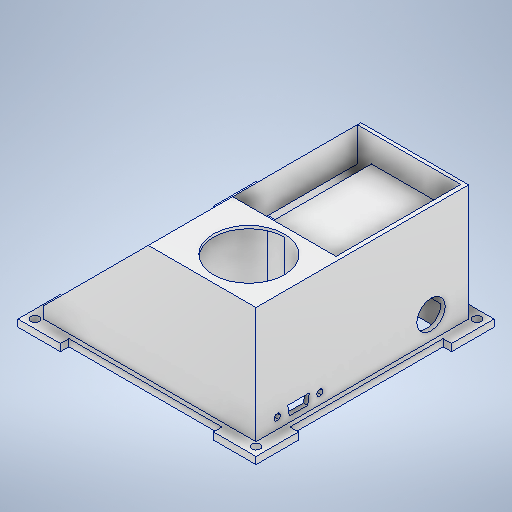
# Autodesk Inventor part: upper half second trial
Saved by Autodesk Inventor 2025 (Build 290162000, 162)
## iProperties
Created: 2024-04-12
Part Number: upper half second trial
Material: Aluminum 6061
Document SubType Name: Modeling
Designer: mahal
Density: 2.7 g/cm^3
Appearance: Aluminum - Flat
Mass: 980.83 g
Surface Area: 1659.79 cm^2
Volume: 363.27 cm^3
Author: mahal
Autodesk Inventor part; units mm, degrees
sketch "Sketch1" plane through (0, 0, 0) normal (0, 1, 0) x (-1, 0, 0)
  line L0 (75, 75) -> (-75, 75)
  line L1 (-75, 75) -> (-75, -75)
  line L2 (-75, -75) -> (75, -75)
  line L3 (75, -75) -> (75, 75)
  line L4 (75, 75) -> (-75, -75) construction
  line L5 (-75, 75) -> (75, -75) construction
  point P0 (0, 0)
  dimension "d0" = 150
  dimension "d1" = 150
  constraints: 12 end point, 2 midpoint, 2 parallel, 1 horizontal, 1 perpendicular
  measures "d0" distance of L2.end L1.end
  measures "d1" distance of L1.end L0.end
extrude "Extrusion1" add sketch "Sketch1" along normal blind 110
ref_plane "Work Plane1" through (0, 0, 0) normal (0, -1, 0) x (1, 0, 0)
sketch "Sketch2" plane through (0, 0, 0) normal (0, -1, 0) x (1, 0, 0)
  line L0 (72, 72) -> (-72, 72)
  line L1 (-72, 72) -> (-72, -72)
  line L2 (-72, -72) -> (72, -72)
  line L3 (72, -72) -> (72, 72)
  line L4 (72, 72) -> (-72, -72) construction
  line L5 (-72, 72) -> (72, -72) construction
  line L6 (72, 72) -> (3, 72)
  line L7 (3, 72) -> (3, 18)
  line L8 (3, 18) -> (72, 18)
  line L9 (72, 18) -> (72, 72)
  line L10 (72, 18) -> (3, 18)
  line L11 (3, 18) -> (3, 14)
  line L12 (3, 14) -> (72, 14)
  line L13 (72, 14) -> (72, 18)
  point P0 (0, 0)
  dimension "d5" = 144
  dimension "d6" = 144
  dimension "d7" = 69
  dimension "d8" = 54
  dimension "d9" = 4
  constraints: 28 end point, 6 parallel, 3 horizontal, 3 perpendicular, 2 midpoint
  measures "d5" distance of L2.end L1.end
  measures "d6" distance of L1.end L0.end
  measures "d7" distance of L8.end L7.end
  measures "d8" distance of L7.end L6.end
  measures "d9" distance of L11.end L10.end
extrude "Extrusion2" cut sketch "Sketch2" against normal blind 5 contours L3 L8 L7 L0
ref_plane "Work Plane2" through (0, 5, 0) normal (0, -1, 0) x (1, 0, 0)
sketch "Sketch4" plane through (0, 5, 0) normal (0, -1, 0) x (1, 0, 0)
  line L0 (72, 18) -> (3, 18)
  line L1 (3, 18) -> (3, 72)
  line L2 (3, 72) -> (72, 72)
  line L3 (72, 72) -> (72, 18)
  line L4 (72, 18) -> (67, 18)
  line L5 (67, 18) -> (67, 25)
  line L6 (67, 25) -> (72, 25)
  line L7 (72, 25) -> (72, 18)
  line L8 (72, 72) -> (67, 72)
  line L9 (67, 72) -> (67, 65)
  line L10 (67, 65) -> (72, 65)
  line L11 (72, 72) -> (72, 65)
  line L12 (67, 18) -> (13, 18)
  line L13 (13, 18) -> (13, 72)
  line L14 (67, 72) -> (13, 72)
  point P0 (0, 0)
  dimension "d13" = 69
  dimension "d14" = 54
  dimension "d15" = 5
  dimension "d16" = 7
  dimension "d17" = 5
  dimension "d18" = 7
  dimension "d19" = 54
  constraints: 30 end point, 6 perpendicular, 4 parallel, 4 point on line, 2 horizontal, 1 collinear
  measures "d13" distance of L1.end L2.end
  measures "d14" distance of L0.end L1.end
  measures "d15" distance of L5.end L6.end
  measures "d16" distance of L4.end L5.end
  measures "d17" distance of L2.end L8.end
  measures "d18" distance of L8.end L9.end
  measures "d19" distance of L4.end L12.end
extrude "Extrusion3" cut sketch "Sketch4" against normal blind 5 contours L0 L13 L2 L9 L10 L3 L6 L5 | L0 L1 L2 L13
ref_plane "Work Plane3" through (0, 10, 0) normal (0, -1, 0) x (1, 0, 0)
sketch "Sketch5" plane through (0, 10, 0) normal (0, -1, 0) x (1, 0, 0)
  line L0 (67, 18) -> (3, 18) projected
  line L1 (67, 18) -> (3, 18)
  line L2 (3, 18) -> (3, 72)
  line L3 (3, 72) -> (67, 72)
  line L4 (67, 72) -> (67, 18)
  line L5 (67, 18) -> (65, 18)
  line L6 (65, 18) -> (65, 20)
  circle A0 centre (65, 20) radius 1
  line L7 (35, 18) -> (35, 24.7965)
  line L8 (67, 45) -> (56.8773, 45)
  circle A1 centre (65, 70) radius 1
  line L9 (72, 25) -> (67, 25) projected
  line L10 (67, 25) -> (72, 25)
  line L11 (67, 65) -> (72, 65) projected
  line L12 (72, 25) -> (72, 65)
  line L13 (72, 65) -> (67, 65)
  line L14 (67, 72) -> (13, 72)
  line L15 (13, 72) -> (40, 72)
  line L16 (40, 72) -> (40, 60.5837)
  circle A2 centre (15, 70) radius 1
  circle A3 centre (15, 20) radius 1
  point P0 (0, 0)
  dimension "d23" = 2
  dimension "d24" = 2
  dimension "d25" = 2
  dimension "d148" = 54
  dimension "d149" = 27
  constraints: 28 end point, 5 perpendicular, 4 centre point, 3 equal length, 3 midpoint, 3 symmetric about line, 2 horizontal, 2 point on line, 1 coincident, 1 vertical, 3 other
  measures "d23" distance of L0.start L5.end
  measures "d24" distance of L5.end L6.end
  measures "d25" diameter of A0
  measures "d148" distance of L3.end L14.end
  measures "d149" distance of L14.end L15.end
extrude "Extrusion4" cut sketch "Sketch5" against normal blind 5 contours A0 | A1 | A2 | A3
sketch "Sketch6" plane through (0, 10, 0) normal (0, -1, 0) x (1, 0, 0)
  line L0 (72, 25) -> (67, 25) projected
  line L1 (67, 25) -> (67, 65) projected
  line L2 (67, 25) -> (67, 65)
  line L3 (67, 45) -> (40, 45)
  line L4 (40, 45) -> (28, 45)
  arc A0 (40, 20) -> (40, 70) centre (40, 45) ccw
  arc A1 (28, 70) -> (28, 20) centre (28, 45) ccw
  line L5 (40, 20) -> (28, 20)
  line L6 (67, 18) -> (3, 18) projected
  line L7 (40, 70) -> (28, 70)
  line L8 (67, 25) -> (55, 25)
  line L9 (72, 65) -> (72, 25) projected
  line L10 (67, 65) -> (55, 65)
  point P0 (0, 0)
  dimension "d28" = 27
  dimension "d29" = 12
  constraints: 14 end point, 6 point on circle, 2 centre point, 2 coincident, 2 horizontal, 2 parallel, 2 tangent, 1 midpoint, 1 perpendicular, 1 vertical
  measures "d28" distance of L3.start L3.end
  measures "d29" distance of L3.end L4.end
extrude "Extrusion5" cut sketch "Sketch6" against normal blind 75
sketch "Sketch7" plane through (0, 0, 0) normal (0, -1, 0) x (1, 0, 0)
  line L0 (72, 18) -> (3, 18)
  line L1 (3, 18) -> (3, 15.5)
  line L2 (3, 15.5) -> (72, 15.5)
  line L3 (72, 15.5) -> (72, 18)
  line L4 (72, 15.5) -> (3, 15.5)
  line L5 (3, 15.5) -> (3, -72.5)
  line L6 (3, -72.5) -> (72, -72.5)
  line L7 (72, -72.5) -> (72, 15.5)
  point P0 (0, 0)
  dimension "d34" = 2.5
  dimension "d35" = 69
  dimension "d36" = 88
  constraints: 16 end point, 4 parallel, 2 horizontal, 2 perpendicular
  measures "d34" distance of L1.end L0.end
  measures "d35" distance of L6.end L5.end
  measures "d36" distance of L5.end L4.end
extrude "Extrusion6" cut sketch "Sketch7" against normal blind 5 contours L7 L6 L5 L2
ref_plane "Work Plane4" through (0, 5, 0) normal (0, -1, 0) x (1, 0, 0)
sketch "Sketch8" plane through (0, 5, 0) normal (0, -1, 0) x (1, 0, 0)
  line L0 (72, 15.5) -> (72, -72.5) projected
  line L1 (72, 15.5) -> (24, 15.5)
  line L2 (3, 15.5) -> (72, 15.5) projected
  line L3 (24, 15.5) -> (24, -72.5)
  line L4 (72, -72.5) -> (3, -72.5) projected
  line L5 (24, 15.5) -> (12, 15.5)
  line L6 (12, 15.5) -> (12, -72.5)
  line L7 (24, -72.5) -> (12, -72.5)
  point P0 (0, 0)
  dimension "d40" = 48
  dimension "d41" = 12
  constraints: 10 end point, 4 point on line, 2 perpendicular, 1 collinear
  measures "d40" distance of L0.start L1.end
  measures "d41" distance of L1.end L5.end
extrude "Extrusion7" cut sketch "Sketch8" against normal blind 54 contours L3 L4 L6 L2
ref_plane "Work Plane5" through (24, 5, 15.5) normal (-1, 0, 0) x (0, 0, 1)
sketch "Sketch10" plane through (24, 5, 15.5) normal (-1, 0, 0) x (0, 0, 1)
  line L0 (-88, 0) -> (-88, 54) projected
  line L1 (-88, 0) -> (-74, 0)
  line L2 (0, 0) -> (-88, 0) projected
  line L3 (-74, 0) -> (-54, 0)
  line L4 (-64, 0) -> (-64, 16)
  circle A0 centre (-64, 16) radius 10
  line L5 (-74, 16) -> (-74, 0)
  line L6 (-88, 0) -> (0, 0) projected
  line L7 (-54, 16) -> (-54, 0)
  point P0 (-15.5, -5)
  point P1 (-54, 0)
  dimension "d47" = 14
  dimension "d48" = 20
  dimension "d49" = 16
  dimension "d50" = 20
  constraints: 10 end point, 2 point on circle, 2 point on line, 2 tangent, 1 centre point, 1 coincident, 1 midpoint, 1 vertical
  measures "d47" distance of L0.start L1.end
  measures "d48" distance of L1.end L3.end
  measures "d49" distance of L4.start L4.end
  measures "d50" diameter of A0
extrude "Extrusion8" cut sketch "Sketch10" against normal up to surface (48 mm away)
ref_plane "Work Plane6" through (72, 0, 15.5) normal (-1, 0, 0) x (0, 0, 1)
sketch "Sketch11" plane through (72, 0, 15.5) normal (-1, 0, 0) x (0, 0, 1)
  line L0 (-74, 5) -> (-88, 5) projected
  line L1 (-54, 5) -> (-74, 5)
  line L2 (-64, 5) -> (-64, 21)
  circle A0 centre (-64, 21) radius 10
  point P0 (-15.5, 0)
  dimension "d54" = 16
  constraints: 4 end point, 1 centre point, 1 coincident, 1 horizontal, 1 midpoint, 1 vertical
  measures "d54" distance of L2.start L2.end
extrude "Extrusion9" cut sketch "Sketch11" against normal up to surface (3 mm away)
sketch "Sketch12" plane through (0, 0, 0) normal (0, -1, 0) x (1, 0, 0)
  line L0 (3, 72) -> (-1, 72)
  line L1 (-75, -75) -> (-75, 75) projected
  line L2 (-75, -75) -> (-71, -75)
  line L3 (75, -75) -> (-75, -75) projected
  line L4 (-1, 72) -> (-71, 72)
  line L5 (-71, 72) -> (-71, -72.5)
  line L6 (-71, -72.5) -> (-1, -72.5)
  line L7 (-1, -72.5) -> (-1, 72)
  point P0 (0, 0)
  dimension "d57" = 4
  dimension "d58" = 4
  constraints: 12 end point, 2 horizontal, 2 parallel, 1 perpendicular, 1 point on line
  measures "d57" distance of L0.start L0.end
  measures "d58" distance of L1.start L2.end
extrude "Extrusion10" cut sketch "Sketch12" against normal up to surface (110 mm away)
ref_plane "Work Plane7" through (-75, 0, 75) normal (0, 0, 1) x (1, 0, 0)
ref_plane "Work Plane8" through (-1, 0, -72.5) normal (-1, 0, 0) x (0, 0, 1)
sketch "Sketch14" plane through (-1, 0, -72.5) normal (-1, 0, 0) x (0, 0, 1)
  line L0 (88, 0) -> (88, 5) projected
  line L1 (-2.5, 110) -> (0, 110) projected
  line L2 (88, 0) -> (0, 0)
  line L3 (0, 0) -> (0, 110)
  line L4 (0, 110) -> (88, 110)
  line L5 (88, 110) -> (88, 0)
  point P0 (72.5, 0)
  constraints: 8 end point, 2 parallel, 1 horizontal, 1 perpendicular
extrude "Extrusion12" cut sketch "Sketch14" against normal blind 10
ref_plane "Work Plane9" through (72, 0, 72) normal (-1, 0, 0) x (0, 0, 1)
sketch "Sketch15" plane through (72, 0, 72) normal (-1, 0, 0) x (0, 0, 1)
  line L0 (-7, 5) -> (-7, 10) projected
  line L1 (-47, 5) -> (-47, 10) projected
  line L2 (-7, 20) -> (-47, 20)
  line L3 (-27, 20) -> (-27, 16.019)
  line L4 (-27, 16.019) -> (-27, 8.979)
  line L5 (-27, 8.979) -> (-20.4672, 8.979)
  line L6 (-19.3975, 16.019) -> (-20.4672, 8.979)
  line L7 (-19.3975, 16.019) -> (-12.2767, 16.019) construction
  line L8 (-47, 20) -> (-42, 20)
  line L9 (-42, 20) -> (-42, 12.5)
  line L10 (-43.179, 10.4579) -> (-44.358, 12.5)
  line L11 (-44.358, 12.5) -> (-43.179, 14.5421)
  line L12 (-43.179, 14.5421) -> (-40.821, 14.5421)
  line L13 (-40.821, 14.5421) -> (-39.642, 12.5)
  line L14 (-39.642, 12.5) -> (-40.821, 10.4579)
  line L15 (-40.821, 10.4579) -> (-43.179, 10.4579)
  line L16 (-12, 20) -> (-12, 12.5)
  line L17 (-10.821, 10.4579) -> (-9.642, 12.5)
  line L18 (-9.642, 12.5) -> (-10.821, 14.5421)
  line L19 (-10.821, 14.5421) -> (-13.179, 14.5421)
  line L20 (-13.179, 14.5421) -> (-14.358, 12.5)
  line L21 (-14.358, 12.5) -> (-13.179, 10.4579)
  line L22 (-13.179, 10.4579) -> (-10.821, 10.4579)
  line L23 (-19.3975, 16.019) -> (-27, 16.019)
  line L24 (-27, 8.979) -> (-33.5328, 8.979)
  line L25 (-34.6025, 16.019) -> (-33.5328, 8.979)
  line L26 (-34.6025, 16.019) -> (-27, 16.019)
  point P0 (-72, 0)
  point P1 (-42, 10.4579)
  point P2 (-12, 10.4579)
  dimension "d74" = 98.64
  dimension "d75" = 5
  dimension "d76" = 7.5
  dimension "d77" = 2.358
  constraints: 50 end point, 12 symmetric about line, 4 horizontal, 3 point on line, 2 coincident, 2 midpoint, 2 vertical, 1 equal length, 1 perpendicular, 13 other
  measures "d74" angle of L6 L7
  measures "d75" distance of L2.end L8.end
  measures "d76" distance of L8.end L9.end
  measures "d77" distance of L14.end L10.start
extrude "Extrusion13" cut sketch "Sketch15" against normal up to surface (3 mm away)
ref_plane "Work Plane10" through (0, 110, 0) normal (0, 1, 0) x (1, 0, 0)
sketch "Sketch16" plane through (0, 110, 0) normal (0, 1, 0) x (1, 0, 0)
  line L0 (-75, 75) -> (-75, -75) projected
  line L1 (-75, -75) -> (79.013, -75)
  line L2 (79.013, -75) -> (79.013, 75)
  line L3 (79.013, 75) -> (-75, 75)
  line L4 (-75, 75) -> (-75, -75)
  point P0 (0, 0)
  constraints: 8 end point, 2 parallel, 1 horizontal, 1 perpendicular
extrude "Extrusion14" cut sketch "Sketch16" against normal blind 23
ref_plane "Work Plane11" through (-75, 0, 75) normal (0, 0, 1) x (1, 0, 0)
sketch "Sketch17" plane through (-75, 0, 75) normal (0, 0, 1) x (1, 0, 0)
  line L0 (4, 0) -> (4, 87) projected
  line L1 (4, 87) -> (74, 87) projected
  line L2 (4, 87) -> (74, 87)
  line L3 (74, 87) -> (4, 17)
  line L4 (4, 0) -> (4, 87) projected
  line L5 (4, 17) -> (4, 85.4864)
  line L6 (0, 0) -> (0, 87) projected
  line L7 (4, 17) -> (0, 13)
  line L8 (0, 87) -> (0, 13)
  line L9 (0, 87) -> (4, 87)
  point P0 (75, 0)
  dimension "d84" = 45
  constraints: 12 end point, 3 point on line, 2 collinear, 1 parallel
  measures "d84" angle of L2 L3
extrude "Extrusion15" cut sketch "Sketch17" against normal up to surface (150 mm away)
ref_plane "Work Plane12" through (0, 5, 0) normal (0, -1, 0) x (1, 0, 0)
sketch "Sketch18" plane through (0, 5, 0) normal (0, -1, 0) x (1, 0, 0)
  line L0 (72, -72.5) -> (26, -72.5)
  line L1 (26, -72.5) -> (26, -60.5)
  line L2 (26, -60.5) -> (72, -60.5)
  line L3 (72, -60.5) -> (72, -72.5)
  line L4 (72, 15.5) -> (72, -38.5) projected
  line L5 (72, 15.5) -> (26, 15.5)
  line L6 (26, 15.5) -> (26, -36.5)
  line L7 (26, -36.5) -> (72, -36.5)
  line L8 (72, -36.5) -> (72, 15.5)
  point P0 (0, 0)
  dimension "d88" = 46
  dimension "d89" = 12
  dimension "d90" = 52
  constraints: 16 end point, 4 parallel, 2 horizontal, 2 perpendicular, 1 point on line
  measures "d88" distance of L1.end L2.end
  measures "d89" distance of L0.end L1.end
  measures "d90" distance of L6.end L5.end
extrude "Extrusion16" cut sketch "Sketch18" against normal up to surface (82 mm away)
ref_plane "Work Plane13" through (26, 87, -36.5) normal (0, 0, 1) x (1, 0, 0)
sketch "Sketch19" plane through (26, 87, -36.5) normal (0, 0, 1) x (1, 0, 0)
  line L0 (0, -82) -> (0, 0) projected
  line L1 (0, 0) -> (46, 0)
  line L2 (46, 0) -> (46, -54)
  line L3 (46, -54) -> (0, -54)
  line L4 (0, -54) -> (0, 0)
  point P0 (-26, -87)
  dimension "d94" = 54
  constraints: 8 end point, 2 parallel, 1 horizontal, 1 perpendicular
  measures "d94" distance of L1.end L2.end
extrude "Extrusion17" cut sketch "Sketch19" against normal up to surface (24 mm away)
ref_plane "Work Plane14" through (9, 0, -72.5) normal (-1, 0, 0) x (0, 0, 1)
sketch "Sketch20" plane through (9, 0, -72.5) normal (-1, 0, 0) x (0, 0, 1)
  line L0 (0, 5) -> (0, 87) projected
  line L1 (88, 87) -> (88, 5) projected
  line L2 (0, 87) -> (88, 87)
  line L3 (88, 87) -> (88, 65)
  line L4 (88, 65) -> (0, 65)
  line L5 (0, 65) -> (0, 87)
  point P0 (72.5, 0)
  dimension "d98" = 22
  constraints: 8 end point, 2 parallel, 1 horizontal, 1 perpendicular, 1 point on line
  measures "d98" distance of L2.end L3.end
extrude "Extrusion18" cut sketch "Sketch20" against normal up to surface (17 mm away)
ref_plane "Work Plane15" through (9, 65, -72.5) normal (0, 1, 0) x (1, 0, 0)
sketch "Sketch21" plane through (9, 65, -72.5) normal (0, 1, 0) x (1, 0, 0)
  line L0 (63, 0) -> (0, 0)
  line L1 (0, 0) -> (0, -88)
  line L2 (0, -88) -> (63, -88)
  line L3 (63, -88) -> (63, 0)
  point P0 (-9, -72.5)
  constraints: 8 end point, 2 parallel, 1 horizontal, 1 perpendicular
extrude "Extrusion19" add sketch "Sketch21" along normal blind 3
ref_plane "Work Plane16" through (0, 87, 0) normal (0, 1, 0) x (1, 0, 0)
sketch "Sketch22" plane through (0, 87, 0) normal (0, 1, 0) x (1, 0, 0)
  line L0 (67, -65) -> (67, -25) projected
  line L1 (67, -25) -> (67, -65)
  line L2 (67, -45) -> (40, -45)
  circle A0 centre (40, -45) radius 25
  line L3 (28, -70) -> (40, -70) projected
  point P0 (0, 0)
  dimension "d105" = 27
  constraints: 4 end point, 2 horizontal, 1 coincident, 1 midpoint, 1 vertical, 1 vertical alignment, 1 other
  measures "d105" distance of L2.start L2.end
extrude "Extrusion20" cut sketch "Sketch22" against normal up to surface (2 mm away)
ref_plane "Work Plane17" through (-1, 0, 72) normal (0, 0, -1) x (-1, 0, 0)
sketch "Sketch23" plane through (-1, 0, 72) normal (0, 0, -1) x (-1, 0, 0)
  line L0 (0, 0) -> (0, 87) projected
  line L1 (0, 87) -> (0, 63)
  line L2 (0, 63) -> (70, -7)
  line L3 (70, 0) -> (70, 17) projected
  line L4 (70, -7) -> (70, 17)
  line L5 (70, 17) -> (0, 87)
  point P0 (-1, 0)
  dimension "d109" = 24
  dimension "d110" = 135
  constraints: 8 end point, 2 parallel, 2 point on line
  measures "d109" distance of L0.end L1.end
  measures "d110" angle of L2 L1
extrude "Extrusion21" add sketch "Sketch23" along normal up to surface (144.5 mm away)
ref_plane "Work Plane18" through (-66.5, -2.5, 72) normal (0.7071068, -0.7071068, 0) x (-0.7071068, -0.7071068, 0)
sketch "Sketch24" plane through (-66.5, -2.5, 72) normal (0.7071068, -0.7071068, 0) x (-0.7071068, -0.7071068, 0)
  line L0 (-92.0916, 97) -> (-48.7904, 122)
  line L1 (-48.7904, 122) -> (-5.4891, 97)
  line L2 (-5.4891, 97) -> (-5.4891, 47)
  line L3 (-5.4891, 47) -> (-48.7904, 22)
  line L4 (-48.7904, 22) -> (-92.0916, 47)
  line L5 (-92.0916, 47) -> (-92.0916, 97)
  point P0 (-48.7904, 72)
  point P1 (-48.7904, 72)
  dimension "d114" = 50
  constraints: 12 end point, 1 coincident, 13 other
  measures "d114" distance of L4.end L0.start
extrude "Extrusion22" cut sketch "Sketch24" against normal blind 12
ref_plane "Work Plane19" through (-74.9853, 5.9853, 72) normal (0.7071068, -0.7071068, 0) x (0, 0, -1)
sketch "Sketch25" plane through (-74.9853, 5.9853, 72) normal (0.7071068, -0.7071068, 0) x (0, 0, -1)
  circle A0 centre (72, 48.7904) radius 17.5
  dimension "d118" = 35
  constraints: 1 centre point, 1 coincident
  measures "d118" diameter of A0
extrude "Extrusion23" cut sketch "Sketch25" against normal up to surface (4.9706 mm away)
ref_plane "Work Plane20" through (-74.9853, 5.9853, 72) normal (0.7071068, -0.7071068, 0) x (0, 0, -1)
sketch "Sketch26" plane through (-74.9853, 5.9853, 72) normal (0.7071068, -0.7071068, 0) x (0, 0, -1)
  line L0 (47, 92.0916) -> (97, 92.0916) projected
  line L1 (47, 92.0916) -> (50, 86.8955)
  line L2 (47, 92.0916) -> (53, 92.0916) construction
  circle A0 centre (50, 86.8955) radius 2.5
  line L3 (122, 48.7904) -> (97, 5.4891) projected
  line L4 (122, 48.7904) -> (116, 48.7904)
  circle A1 centre (116, 48.7904) radius 2.5
  line L5 (47, 5.4891) -> (22, 48.7904) projected
  line L6 (47, 5.4891) -> (50, 10.6853)
  line L7 (47, 5.4891) -> (53, 5.4891) construction
  circle A2 centre (50, 10.6853) radius 2.5
  point P0 (72, 48.7904)
  dimension "d122" = 6
  dimension "d123" = 60
  dimension "d124" = 5
  dimension "d125" = 6
  dimension "d126" = 5
  dimension "d127" = 60
  dimension "d128" = 5
  constraints: 10 end point, 3 centre point, 3 coincident, 3 horizontal, 2 equal length
  measures "d122" distance of L0.start L1.end
  measures "d123" angle of L1 L2
  measures "d124" diameter of A0
  measures "d125" distance of L3.start L4.end
  measures "d126" diameter of A1
  measures "d127" angle of L7 L6
  measures "d128" diameter of A2
extrude "Extrusion24" cut sketch "Sketch26" against normal blind 4
ref_plane "Work Plane21" through (-71, -7, 72) normal (0.7071068, -0.7071068, 0) x (-0.7071068, -0.7071068, 0)
sketch "Sketch27" plane through (-71, -7, 72) normal (0.7071068, -0.7071068, 0) x (-0.7071068, -0.7071068, 0)
  line L0 (-55.1543, 122) -> (-11.8531, 97) projected
  line L1 (-11.8531, 100) -> (-11.8531, 144.5)
  line L2 (-98.9949, 144.5) -> (-9.8995, 144.5) projected
  line L3 (-11.8531, 97) -> (35.6469, 97) construction
  line L4 (-11.8531, 144.5) -> (-97.8531, 144.5)
  line L5 (-97.8531, 144.5) -> (-98.4556, 97)
  line L6 (-98.4556, 97) -> (-98.4175, 99.9998)
  line L7 (-98.4175, 99.9998) -> (-55.1351, 124.9889)
  line L8 (-98.4556, 97) -> (-55.1543, 122) projected
  line L9 (-11.8531, 97) -> (-11.8531, 100)
  line L10 (-11.8531, 100) -> (-55.1351, 124.9889)
  line L11 (-11.8531, 97) -> (-11.8531, 47) projected
  line L12 (-11.8531, 97) -> (-11.8531, 47)
  line L13 (-11.8531, 72) -> (-35.2679, 72)
  line L14 (-11.8531, 44) -> (-11.8531, -0.5)
  line L15 (-98.9949, -0.5) -> (-9.8995, -0.5)
  line L16 (-97.8531, -0.5) -> (-98.4556, 47)
  line L17 (-98.4175, 44.0002) -> (-55.1351, 19.0111)
  line L18 (-11.8531, 44) -> (-55.1351, 19.0111)
  point P0 (-55.1543, 72)
  dimension "d132" = 90
  dimension "d133" = 86
  dimension "d134" = 3
  dimension "d135" = 3
  constraints: 30 end point, 8 symmetric about line, 4 point on line, 2 horizontal, 2 parallel, 1 collinear, 1 midpoint, 1 perpendicular
  measures "d132" angle of L3 L1
  measures "d133" distance of L1.end L4.end
  measures "d134" distance of L5.end L6.end
  measures "d135" distance of L1.start L0.end
extrude "Extrusion25" cut sketch "Sketch27" against normal up to surface (12 mm away) contours L10 L7 L5 L2 L1 | L14 L15 L16 L17 L18
ref_plane "Work Plane22" through (9, 0, -72.5) normal (-1, 0, 0) x (0, 0, 1)
sketch "Sketch28" plane through (9, 0, -72.5) normal (-1, 0, 0) x (0, 0, 1)
  line L0 (88, 5) -> (88, 59) projected
  line L1 (88, 5) -> (0, 5)
  line L2 (0, 5) -> (0, 59)
  line L3 (0, 59) -> (88, 59)
  line L4 (88, 59) -> (88, 5)
  line L5 (88, 5) -> (88, 9.912)
  line L6 (88, 68) -> (88, 5) projected
  line L7 (88, 5) -> (92.912, 5) construction
  line L8 (88, 9.912) -> (83.954, 9.912)
  circle A0 centre (83.954, 9.912) radius 2
  line L9 (44, 5) -> (44, 9.912)
  line L10 (88, 36.5) -> (81.954, 36.5)
  line L11 (88, 36.5) -> (94.046, 36.5) construction
  circle A1 centre (4.046, 9.912) radius 2
  circle A2 centre (83.954, 63.088) radius 2
  circle A3 centre (4.046, 63.088) radius 2
  point P0 (72.5, 0)
  dimension "d139" = 88
  dimension "d140" = 54
  dimension "d141" = 4.912
  dimension "d142" = 90
  dimension "d143" = 4.046
  dimension "d144" = 4
  dimension "d145" = 180
  constraints: 20 end point, 4 centre point, 3 horizontal, 3 symmetric about line, 2 equal length, 2 midpoint, 2 parallel, 2 perpendicular, 1 coincident, 1 collinear, 1 vertical, 3 other
  measures "d139" distance of L2.end L3.end
  measures "d140" distance of L1.end L2.end
  measures "d141" distance of L0.start L5.end
  measures "d142" angle of L7 L5
  measures "d143" distance of L5.end L8.end
  measures "d144" diameter of A0
  measures "d145" angle of L10 L11
extrude "Extrusion26" cut sketch "Sketch28" against normal up to surface (3 mm away) contours A0 | A1 | A2 | A3
ref_plane "Work Plane23" through (-1, 0, 72) normal (0, 0, 1) x (1, 0, 0)
sketch "Sketch29" plane through (-1, 0, 72) normal (0, 0, 1) x (1, 0, 0)
  line L0 (-63, 0) -> (-61.6186, 1.3814) projected
  line L1 (-70, 0) -> (-63, 0)
  line L2 (-63, 0) -> (-70, -7)
  line L3 (-70, -7) -> (-70, 0)
  point P0 (1, 0)
  constraints: 6 end point, 1 collinear, 1 horizontal, 1 perpendicular
extrude "Extrusion27" cut sketch "Sketch29" against normal up to surface (144.5 mm away)
ref_plane "Work Plane24" through (0, 0, 0) normal (0, -1, 0) x (1, 0, 0)
sketch "Sketch30" plane through (0, 0, 0) normal (0, -1, 0) x (1, 0, 0)
  line L0 (78, 78) -> (-78, 78)
  line L1 (-78, 78) -> (-78, -78)
  line L2 (-78, -78) -> (78, -78)
  line L3 (78, -78) -> (78, 78)
  line L4 (78, 78) -> (-78, -78) construction
  line L5 (-78, 78) -> (78, -78) construction
  line L6 (78, 78) -> (84, 78)
  line L7 (84, 78) -> (84, 84)
  line L8 (84, 84) -> (78, 84)
  line L9 (78, 84) -> (78, 78)
  line L10 (84, 78) -> (78, 78)
  line L11 (78, 78) -> (78, 54)
  line L12 (78, 54) -> (84, 54)
  line L13 (84, 54) -> (84, 78)
  line L14 (78, 84) -> (54, 84)
  line L15 (54, 84) -> (54, 78)
  line L16 (54, 78) -> (78, 78)
  line L17 (78, 78) -> (78, 84)
  line L18 (78, 0) -> (50.5525, 0)
  line L19 (0, 78) -> (0, 48.979)
  line L20 (3, 45) -> (3, 72) projected
  line L21 (84, -78) -> (84, -84)
  line L22 (84, -84) -> (78, -84)
  line L23 (78, -84) -> (78, -78)
  line L24 (78, -54) -> (84, -54)
  line L25 (84, -54) -> (84, -78)
  line L26 (78, -84) -> (54, -84)
  line L27 (54, -84) -> (54, -78)
  line L28 (78, -78) -> (78, -84)
  line L29 (-78, 78) -> (-84, 78)
  line L30 (-84, 84) -> (-78, 84)
  line L31 (-78, 84) -> (-78, 78)
  line L32 (-84, 78) -> (-78, 78)
  line L33 (-78, 54) -> (-84, 54)
  line L34 (-84, 54) -> (-84, 78)
  line L35 (-78, 84) -> (-54, 84)
  line L36 (-54, 84) -> (-54, 78)
  line L37 (-78, 78) -> (-78, 84)
  line L38 (-54, -84) -> (-54, -78)
  line L39 (-78, -84) -> (-54, -84)
  line L40 (-84, -78) -> (-84, -84)
  line L41 (-84, -84) -> (-78, -84)
  line L42 (-78, -54) -> (-84, -54)
  line L43 (-84, -54) -> (-84, -78)
  line L44 (-84, 78) -> (-84, 84)
  line L45 (-75, -75) -> (-75, 75) projected
  line L46 (75, 75) -> (-75, 75)
  line L47 (-75, 75) -> (-75, -75)
  line L48 (-75, -75) -> (75, -75)
  line L49 (75, -75) -> (75, 75)
  line L50 (75, 75) -> (-75, -75) construction
  line L51 (-75, 75) -> (75, -75) construction
  point P0 (0, 0)
  dimension "d154" = 156
  dimension "d155" = 156
  dimension "d156" = 6
  dimension "d157" = 6
  dimension "d158" = 24
  dimension "d159" = 24
  constraints: 100 end point, 26 symmetric about line, 11 parallel, 6 horizontal, 6 midpoint, 5 perpendicular, 2 point on line, 1 vertical
  measures "d154" distance of L2.end L1.end
  measures "d155" distance of L1.end L0.end
  measures "d156" distance of L8.end L7.end
  measures "d157" distance of L7.end L6.end
  measures "d158" distance of L11.end L10.end
  measures "d159" distance of L16.end L15.end
extrude "Extrusion28" add sketch "Sketch30" against normal blind 5 contours L3 L18 L49 L46 L19 L0 | L6 L13 L12 L3 | L9 L8 L7 L6 | L0 L15 L14 L9 | L19 L46 L45 L48 L49 L18 L3 L2 L1 L0 | L0 L31 L35 L36 | L24 L25 L21 L22 L23 L3 | L1 L33 L34 L29 | L29 L44 L30 L31 | L23 L26 L27 L2 | L1 L2 L38 L39 L41 L40 L43 L42
ref_plane "Work Plane25" through (0, 10, 0) normal (0, -1, 0) x (1, 0, 0)
sketch "Sketch31" plane through (0, 10, 0) normal (0, -1, 0) x (1, 0, 0)
  line L0 (72, 65) -> (72, 51.6879) projected
  line L1 (72, 65) -> (67, 65)
  line L2 (67, 65) -> (67, 25)
  line L3 (67, 25) -> (72, 25)
  line L4 (72, 25) -> (72, 65)
  point P0 (0, 0)
  constraints: 8 end point, 2 parallel, 1 horizontal, 1 perpendicular
extrude "Extrusion29" cut sketch "Sketch31" against normal blind 10
sketch "Sketch32" plane through (0, 0, 0) normal (0, -1, 0) x (1, 0, 0)
  line L0 (12, -72.5) -> (12, 15.5) projected
  line L1 (12, 15.5) -> (12, 18)
  line L2 (67, 18) -> (3, 18) projected
  line L3 (12, 15.5) -> (-1, 15.5)
  line L4 (-1, 15.5) -> (-1, 36.8215)
  line L5 (-1, 36.8215) -> (3, 36.8215)
  line L6 (3, 18) -> (3, 72) projected
  line L7 (3, 36.8215) -> (12, 18)
  line L8 (-1, 72) -> (-1, 15.5) projected
  line L9 (-1, 43.75) -> (3, 43.75)
  line L10 (12, 72) -> (12, 69.5)
  line L11 (12, 72) -> (-1, 72)
  line L12 (-1, 72) -> (-1, 50.6785)
  line L13 (-1, 50.6785) -> (3, 50.6785)
  line L14 (3, 50.6785) -> (12, 69.5)
  point P0 (0, 0)
  dimension "d165" = 4
  constraints: 22 end point, 5 symmetric about line, 3 point on line, 2 horizontal, 2 perpendicular, 1 midpoint, 1 vertical
  measures "d165" distance of L4.end L5.end
extrude "Extrusion30" cut sketch "Sketch32" against normal blind 80 contours L3 L4 L5 L6 L2 L1 | L2 L6 L7
sketch "Sketch33" plane through (0, 0, 0) normal (0, -1, 0) x (1, 0, 0)
  line L0 (84, 84) -> (54, 84) projected
  line L1 (84, 84) -> (78, 84)
  line L2 (78, 84) -> (78, 78)
  line L3 (78, 78) -> (84, 78)
  line L4 (84, 78) -> (84, 84)
  circle A0 centre (78, 78) radius 3
  line L5 (78, 0) -> (48.867, 0)
  line L6 (72, 15.5) -> (72, -72.5) projected
  line L7 (-54, 78) -> (54, 78) projected
  line L8 (0, 78) -> (0, 6.3914)
  line L9 (-1, 72) -> (-1, 36.8215) projected
  circle A1 centre (78, -78) radius 3
  circle A2 centre (-78, 78) radius 3
  circle A3 centre (-78, -78) radius 3
  point P0 (0, 0)
  dimension "d168" = 6
  dimension "d169" = 6
  dimension "d170" = 6
  constraints: 12 end point, 4 centre point, 3 parallel, 3 symmetric about line, 2 perpendicular, 1 coincident, 1 horizontal, 1 midpoint, 3 other
  measures "d168" distance of L3.end L2.end
  measures "d169" distance of L2.end L1.end
  measures "d170" diameter of A0
extrude "Extrusion31" cut sketch "Sketch33" against normal up to surface (5 mm away) contours A0 L3 L2 | L2 L3 A0 | A1 | A2 | A3
body "Solid1"
